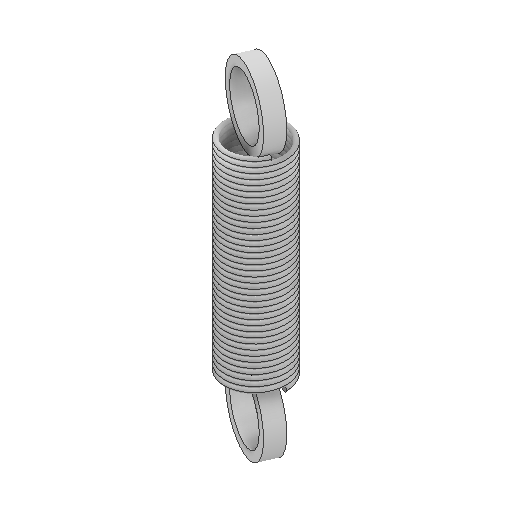
# Autodesk Inventor part: Spring PROP
Saved by Autodesk Inventor 2025 (Build 290162010, 162A)
## iProperties
Created: 2024-12-11
Part Number: Spring PROP
Material: Generic
Document SubType Name: Modeling
Designer: ALEXANDERNICHOLS
Density: 1 g/cm^3
Appearance: Default
Author: ALEXANDERNICHOLS
Autodesk Inventor part; units mm, degrees
ref_plane "YZ Plane" through (0, 0, 0) normal (1, 0, 0) x (0, 1, 0)
ref_plane "XZ Plane" through (0, 0, 0) normal (0, 1, 0) x (-1, 0, 0)
ref_plane "XY Plane" through (0, 0, 0) normal (0, 0, 1) x (1, 0, 0)
sketch "Sketch1" plane through (0, 0, 0) normal (0, 0, 1) x (1, 0, 0)
  line L0 (0, 0) -> (0, 29.6672)
  circle A0 centre (4.1402, 0) radius 0.3175
  dimension "d0" = 29.6672
  dimension "d1" = 0.635
  dimension "d2" = 4.1402
  constraints: 2 end point, 1 centre point, 1 vertical
  measures "d0" distance of L0.start L0.end
  measures "d1" diameter of A0
  measures "d2" distance from line of L0 A0.centre
coil "Coil1" sketch "Sketch1" operation add axis through (0, 0, 0) along (0, 1, 0) pitch 0.762 turns 38.933333 hand right
sketch "Sketch2" plane through (3.7823, 29.6672, 1.684) normal (0.4067, 0, -0.9135) x (-0.9135, 0, -0.4067)
  point P0 (4.1402, -29.6672)
sketch "Sketch3" plane through (3.7823, 29.6672, 1.684) normal (0.4067, 0, -0.9135) x (-0.9135, 0, -0.4067)
  circle A0 centre (4.1402, 4.0117) radius 4.191
  circle A1 centre (4.1402, -34.0883) radius 4.191
  circle A2 centre (4.1402, 4.0117) radius 5.461
  circle A3 centre (4.1402, -34.0883) radius 5.461
  point P0 (4.1402, -29.6672)
  dimension "d11" = 8.382
  dimension "d12" = 8.382
  dimension "d13" = 38.1
  dimension "d14" = 1.27
  dimension "d15" = 1.27
  constraints: 4 centre point, 2 coincident, 1 vertical alignment
  measures "d11" diameter of A0
  measures "d12" diameter of A1
  measures "d13" distance of A0.centre A1.centre
  measures "d14" radial gap between concentric circles of A2 A0
  measures "d15" radial gap between concentric circles of A3 A1
extrude "Extrusion1" add sketch "Sketch3" along normal mid plane 2.54
equation "\"d4\" = d0"
equation "\"d12\" = d11"
equation "\"d15\" = d14"
body "Solid1"
